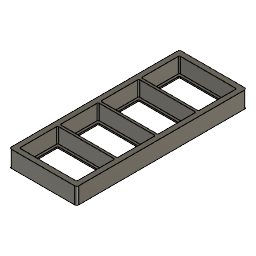
c64_kb_1_5U_grid (Autodesk Fusion 360 design; units mm, degrees)
part number: c64_kb_1_5U_grid
Autodesk Fusion 360 part; units mm, degrees
sketch "Sketch1" plane through (0, 0, 0) normal (0, 0, 1) x (1, 0, 0)
  line L0 (0.5, 0) -> (27.4, 0)
  line L1 (27.9, 0.5) -> (27.9, 18.1)
  line L2 (27.4, 18.6) -> (0.5, 18.6)
  line L3 (0, 18.1) -> (0, 0.5)
  arc A0 (0, 0.5) -> (0.5, 0) centre (0.5, 0.5) ccw
  arc A1 (27.4, 0) -> (27.9, 0.5) centre (27.4, 0.5) ccw
  arc A2 (27.9, 18.1) -> (27.4, 18.6) centre (27.4, 18.1) ccw
  arc A3 (0.5, 18.6) -> (0, 18.1) centre (0.5, 18.1) ccw
  line L4 (1.7, 17.4) -> (26.2, 17.4)
  line L5 (26.7, 16.9) -> (26.7, 1.7)
  line L6 (26.2, 1.2) -> (1.7, 1.2)
  line L7 (1.2, 1.7) -> (1.2, 16.9)
  arc A4 (1.7, 17.4) -> (1.2, 16.9) centre (1.7, 16.9) ccw
  arc A5 (26.7, 16.9) -> (26.2, 17.4) centre (26.2, 16.9) ccw
  arc A6 (26.2, 1.2) -> (26.7, 1.7) centre (26.2, 1.7) ccw
  arc A7 (1.2, 1.7) -> (1.7, 1.2) centre (1.7, 1.7) ccw
  line L8 (27.4, 38.4) -> (0.5, 38.4)
  line L9 (0, 37.9) -> (0, 20.3)
  arc A8 (26.2, 21) -> (26.7, 21.5) centre (26.2, 21.5) ccw
  line L10 (1.7, 37.2) -> (26.2, 37.2)
  arc A9 (27.9, 37.9) -> (27.4, 38.4) centre (27.4, 37.9) ccw
  arc A10 (0, 20.3) -> (0.5, 19.8) centre (0.5, 20.3) ccw
  line L11 (1.2, 21.5) -> (1.2, 36.7)
  arc A11 (1.7, 37.2) -> (1.2, 36.7) centre (1.7, 36.7) ccw
  line L12 (27.9, 20.3) -> (27.9, 37.9)
  arc A12 (26.7, 36.7) -> (26.2, 37.2) centre (26.2, 36.7) ccw
  line L13 (0.5, 19.8) -> (27.4, 19.8)
  line L14 (26.2, 21) -> (1.7, 21)
  arc A13 (1.2, 21.5) -> (1.7, 21) centre (1.7, 21.5) ccw
  arc A14 (27.4, 19.8) -> (27.9, 20.3) centre (27.4, 20.3) ccw
  arc A15 (0.5, 38.4) -> (0, 37.9) centre (0.5, 37.9) ccw
  line L15 (26.7, 36.7) -> (26.7, 21.5)
  line L16 (27.4, 58.2) -> (0.5, 58.2)
  line L17 (0, 57.7) -> (0, 40.1)
  arc A16 (26.2, 40.8) -> (26.7, 41.3) centre (26.2, 41.3) ccw
  line L18 (1.7, 57) -> (26.2, 57)
  arc A17 (27.9, 57.7) -> (27.4, 58.2) centre (27.4, 57.7) ccw
  arc A18 (0, 40.1) -> (0.5, 39.6) centre (0.5, 40.1) ccw
  line L19 (1.2, 41.3) -> (1.2, 56.5)
  arc A19 (1.7, 57) -> (1.2, 56.5) centre (1.7, 56.5) ccw
  line L20 (27.9, 40.1) -> (27.9, 57.7)
  arc A20 (26.7, 56.5) -> (26.2, 57) centre (26.2, 56.5) ccw
  line L21 (0.5, 39.6) -> (27.4, 39.6)
  line L22 (26.2, 40.8) -> (1.7, 40.8)
  arc A21 (1.2, 41.3) -> (1.7, 40.8) centre (1.7, 41.3) ccw
  arc A22 (27.4, 39.6) -> (27.9, 40.1) centre (27.4, 40.1) ccw
  arc A23 (0.5, 58.2) -> (0, 57.7) centre (0.5, 57.7) ccw
  line L23 (26.7, 56.5) -> (26.7, 41.3)
  line L24 (-1.5, 80.5) -> (29.4, 80.5)
  line L25 (30.4, 79.5) -> (30.4, -1.5)
  line L26 (29.4, -2.5) -> (-1.5, -2.5)
  line L27 (-2.5, -1.5) -> (-2.5, 79.5)
  arc A24 (-1.5, 80.5) -> (-2.5, 79.5) centre (-1.5, 79.5) ccw
  arc A25 (30.4, 79.5) -> (29.4, 80.5) centre (29.4, 79.5) ccw
  arc A26 (29.4, -2.5) -> (30.4, -1.5) centre (29.4, -1.5) ccw
  arc A27 (-2.5, -1.5) -> (-1.5, -2.5) centre (-1.5, -1.5) ccw
  line L28 (0, 77.5) -> (0, 59.9)
  arc A28 (1.2, 61.1) -> (1.7, 60.6) centre (1.7, 61.1) ccw
  line L29 (26.2, 60.6) -> (1.7, 60.6)
  arc A29 (0.5, 78) -> (0, 77.5) centre (0.5, 77.5) ccw
  arc A30 (0, 59.9) -> (0.5, 59.4) centre (0.5, 59.9) ccw
  line L30 (27.4, 78) -> (0.5, 78)
  line L31 (1.2, 61.1) -> (1.2, 76.3)
  line L32 (1.7, 76.8) -> (26.2, 76.8)
  arc A31 (1.7, 76.8) -> (1.2, 76.3) centre (1.7, 76.3) ccw
  line L33 (0.5, 59.4) -> (27.4, 59.4)
  arc A32 (26.7, 76.3) -> (26.2, 76.8) centre (26.2, 76.3) ccw
  line L34 (26.7, 76.3) -> (26.7, 61.1)
  arc A33 (27.4, 59.4) -> (27.9, 59.9) centre (27.4, 59.9) ccw
  arc A34 (26.2, 60.6) -> (26.7, 61.1) centre (26.2, 61.1) ccw
  line L35 (27.9, 59.9) -> (27.9, 77.5)
  arc A35 (27.9, 77.5) -> (27.4, 78) centre (27.4, 77.5) ccw
  point P0 (27.9, 0)
  point P1 (0, 18.6)
  point P2 (0, 19.8)
  point P3 (27.9, 19.8)
  point P4 (0, 19.8)
  point P5 (0, 38.4)
  point P6 (0, 39.6)
  point P7 (27.9, 39.6)
  point P8 (0, 39.6)
  point P9 (0, 58.2)
  point P10 (0, 59.4)
  point P11 (0, 78)
  point P12 (0, 59.4)
  point P13 (27.9, 59.4)
  dimension "d7" = 27.9
  dimension "d8" = 18.6
  dimension "d9" = 0.5
  dimension "d10" = 0.5
  dimension "d12" = 0.5
  dimension "d13" = 0.5
  dimension "d14" = 1.2
  dimension "d15" = 1.2
  dimension "d16" = 1.2
  dimension "d17" = 1.2
  dimension "d18" = 0.5
  dimension "d19" = 0.5
  dimension "d20" = 0.5
  dimension "d21" = 0.5
  dimension "d24" = 29.1
  dimension "d25" = 19.8
  dimension "d35" = 1
  dimension "d36" = 1
  dimension "d37" = 1
  dimension "d38" = 1
  dimension "d48" = 19.8
  dimension "d49" = 19.8
  dimension "d53" = 2.5
  dimension "d54" = 2.5
  dimension "d55" = 2.5
  dimension "d56" = 2.5
  dimension "d56" = 2.5
  constraint horizontal L0
  constraint vertical L1
  constraint horizontal L2
  constraint vertical L3
  constraint coincident origin L0
  constraint coincident origin L3
  constraint tangent L0 A0
  constraint tangent L3 A0
  constraint coincident P0 L0
  constraint coincident P0 L1
  constraint tangent L0 A1
  constraint tangent L1 A1
  constraint tangent L1 A2
  constraint tangent L2 A2
  constraint coincident P1 L2
  constraint coincident P1 L3
  constraint tangent L2 A3
  constraint tangent L3 A3
  constraint horizontal L4
  constraint vertical L5
  constraint horizontal L6
  constraint vertical L7
  constraint tangent L4 A4
  constraint tangent L7 A4
  constraint tangent L4 A5
  constraint tangent L5 A5
  constraint tangent L5 A6
  constraint tangent L6 A6
  constraint tangent L6 A7
  constraint tangent L7 A7
  constraint horizontal L24
  constraint vertical L25
  constraint vertical L27
  constraint tangent L24 A24
  constraint tangent L27 A24
  constraint tangent L24 A25
  constraint tangent L25 A25
  constraint tangent L25 A26
  constraint tangent L26 A26
  constraint tangent L26 A27
  constraint tangent L27 A27
  measures "d7" distance of origin P0
  measures "d8" distance of origin P1
  measures "d9" radius of A0
  measures "d10" radius of A1
  measures "d12" radius of A2
  measures "d13" radius of A3
  measures "d14" distance of L2 L4
  measures "d15" distance of L0 L6
  measures "d16" distance of L3 L7
  measures "d17" distance of L1 L5
  measures "d18" radius of A4
  measures "d19" radius of A5
  measures "d20" radius of A6
  measures "d21" radius of A7
  measures "d35" radius of A24
  measures "d36" radius of A25
  measures "d37" radius of A26
  measures "d38" radius of A27
  measures "d53" distance of L27 L28
  measures "d54" distance of L24 L30
  measures "d55" distance of L25 L35
  measures "d56" distance of L0 L26
extrude "Extrude1" add sketch "Sketch1" along normal blind 0.7 contours L0 L1 L2 L3 A0 A1 A2 A3 | L8 L9 A9 A10 L12 L13 A14 A15 | L16 L17 A17 A18 L20 L21 A22 A23 | L28 A29 A30 L30 L33 A33 L35 A35 makes body 1 at (9.8667, 0.4, 0) makes body 2 at (18.0333, 20.2, 0) makes body 3 at (9.8667, 57.8, 0) makes body 4 at (9.8667, 77.6, 0)
extrude "Extrude2" add sketch "Sketch1" along normal blind 8.1 contours L24 L25 L26 L27 A24 A25 A26 A27 bodies 1 4 2 3
equation "width_1_5U = 27.6 mm + tol"
equation "height_1_5U = 18.3 mm + tol"
equation "distx = width_1_5U + 1.2 mm"
equation "disty = height_1_5U + 1.2 mm"
equation "height_dsa = 7.4 mm"
equation "rim = 1.2 mm"
equation "d7 = width_1_5U"
equation "d8 = height_1_5U"
equation "tol = 0.3 mm"
equation "d14 = rim"
equation "d15 = rim"
equation "d16 = rim"
equation "d17 = rim"
equation "d24 = distx"
equation "d25 = disty"
equation "d36 = d35"
equation "hoffs = 0.7 mm"
equation "d40 = hoffs"
equation "d42 = hoffs + height_dsa"
equation "d48 = disty"
equation "d49 = disty"
